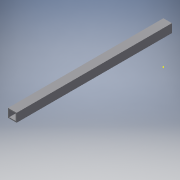
# Autodesk Inventor part: 2018 Bottom Cross Bar
Saved by Autodesk Inventor 2018 (Build 220112000, 112)
## iProperties
Created: 2018-01-26
Part Number: 2018 Bottom Cross Bar
Material: Generic
Document SubType Name: Modeling
Designer: Apple
Density: 1 g/cm^3
Appearance: Default
Author: Apple
Autodesk Inventor part; units mm, degrees
ref_plane "YZ Plane" through (0, 0, 0) normal (1, 0, 0) x (0, 1, 0)
ref_plane "XZ Plane" through (0, 0, 0) normal (0, 1, 0) x (-1, 0, 0)
ref_plane "XY Plane" through (0, 0, 0) normal (0, 0, 1) x (1, 0, 0)
sketch "Sketch1" plane through (0, 0, 0) normal (0, 0, 1) x (1, 0, 0)
  line L0 (-46.6093, 125.5803) -> (-21.2093, 125.5803)
  line L1 (-21.2093, 125.5803) -> (-21.2093, 100.1803)
  line L2 (-21.2093, 100.1803) -> (-46.6093, 100.1803)
  line L3 (-46.6093, 100.1803) -> (-46.6093, 125.5803)
  line L4 (-43.4343, 122.4053) -> (-24.3843, 122.4053)
  line L5 (-24.3843, 122.4053) -> (-24.3843, 103.3553)
  line L6 (-24.3843, 103.3553) -> (-43.4343, 103.3553)
  line L7 (-43.4343, 103.3553) -> (-43.4343, 122.4053)
  point P0 (0, 0)
  dimension "d0" = 25.4
  dimension "d1" = 25.4
  dimension "d2" = 3.175
  constraints: 16 end point, 4 parallel, 2 perpendicular, 1 horizontal, 3 other
  measures "d0" distance of L0.start L0.end
  measures "d1" distance of L0.end L1.end
  measures "d2" distance between parallel lines of L3 L7
extrude "Extrusion1" add sketch "Sketch1" along normal blind 460.375
sketch "Sketch2" plane through (-46.6093, 100.1803, 0) normal (-1, 0, 0) x (0, 0, 1)
  point P0 (0, -100.1803)
sketch "Sketch3" plane through (-46.6093, 100.1803, 0) normal (-1, 0, 0) x (0, 0, 1)
  point P0 (0, -100.1803)
chamfer "Chamfer1" distance 22.225 angle 45 2 edges at (-33.9093, 125.5803, 460.375) (-33.9093, 125.5803, 0)
body "Solid1"
